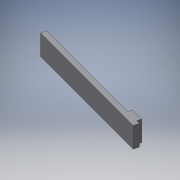
# Autodesk Inventor part: Spring
Saved by Autodesk Inventor 2016 SP2 (Build 200236200, 236)
## iProperties
Created: 2018-09-27
Part Number: Spring
Material: Generisch
Document SubType Name: Modeling
Designer: Nils
Density: 1 g/cm^3
Appearance: Vorgabe
Author: Nils
Autodesk Inventor part; units mm, degrees
ref_plane "YZ Plane" through (0, 0, 0) normal (1, 0, 0) x (0, 1, 0)
ref_plane "XZ Plane" through (0, 0, 0) normal (0, 1, 0) x (-1, 0, 0)
ref_plane "XY Plane" through (0, 0, 0) normal (0, 0, 1) x (1, 0, 0)
sketch "Skizze1" plane through (0, 0, 0) normal (0, 0, 1) x (1, 0, 0)
  line L0 (52.7974, -26.0018) -> (57.627, -27.2959) projected
  line L1 (52.3833, -27.5473) -> (52.7974, -26.0018) projected
  line L2 (57.627, -27.2959) -> (57.2129, -28.8414) projected
  line L3 (58.6618, -29.2296) -> (58.1442, -31.1615) projected
  line L4 (57.2129, -28.8414) -> (58.6618, -29.2296) projected
  line L5 (58.1442, -31.1615) -> (8.882, -17.9617)
  line L6 (8.882, -17.9617) -> (9.3996, -16.0299)
  line L7 (9.3996, -16.0299) -> (52.3833, -27.5473)
  point P0 (0, 0)
  dimension "d0" = 51
  dimension "d2" = 2
  constraints: 6 end point, 1 parallel, 1 perpendicular
  measures "d0" distance of L3.end L5.end
  measures "d2" distance of L5.end L6.end
extrude "Extrusion1" add sketch "Skizze1" against normal blind 8
